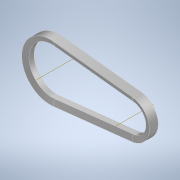
# Autodesk Inventor part: Klapp_Keilriemen
Saved by Autodesk Inventor 2021 (Build 250183000, 183)
## iProperties
CustomPartVersion: 1
Created: 2021-01-13
Part Number: Klapp_Keilriemen
Material: Rubber
Document SubType Name: Modeling
Designer: Jaro Machnow
Density: 0.93 g/cm^3
Appearance: Rubber - Black - Version 1.1
Author: Jaro Machnow
Autodesk Inventor part; units mm, degrees
ref_plane "YZ Plane" through (0, 0, 0) normal (1, 0, 0) x (0, 1, 0)
ref_plane "XZ Plane" through (0, 0, 0) normal (0, 1, 0) x (-1, 0, 0)
sketch "Skizzenpfad" plane through (0, 0, 0) normal (0, 0, 1) x (1, 0, 0)
  arc A0 (-98.3681, 14.911) -> (-98.3681, -14.911) centre (-100, 0) ccw
  arc A1 (-52.9542, -9.9406) -> (-52.9542, 9.9406) centre (-54.0422, 0) ccw
  line L0 (-52.9542, -9.9406) -> (-98.3681, -14.911)
  line L1 (-98.3681, 14.911) -> (-52.9542, 9.9406)
  constraints: 4 end point, 4 point on circle, 2 centre point
ref_plane "Querschnittsebene" through (-98.3681, -14.911, 0) normal (0.9941, 0.1088, 0) x (0, 0, 1)
sketch "Querschnitt" plane through (-98.3681, -14.911, 0) normal (0.9941, 0.1088, 0) x (0, 0, 1)
  line L0 (0, 1.2493) -> (0, -1.7507) construction
  line L1 (-2.1, 0) -> (2.1, 0) construction
  line L2 (-2.5547, 1.2493) -> (2.5547, 1.2493)
  line L3 (2.5547, 1.2493) -> (1.4628, -1.7507)
  line L4 (1.4628, -1.7507) -> (-1.4628, -1.7507)
  line L5 (-1.4628, -1.7507) -> (-2.5547, 1.2493)
  point P0 (0, 0)
  point P1 (0, 0)
  point P2 (0, 0)
  dimension "d0" = 4.2
  dimension "d1" = 1.2493
  dimension "d2" = 40
  dimension "d3" = 3
  constraints: 12 end point, 3 midpoint, 2 parallel, 2 point on line, 1 coincident, 1 perpendicular, 1 vertical, 1 other
  measures "d0" distance of L1.start L1.end
  measures "d1" distance between parallel lines of L2 L1
  measures "d2" angle of L5 L3
  measures "d3" distance between parallel lines of L4 L2
sweep "Riemen" add profiles "Querschnitt" path "Skizzenpfad"
equation "\"d0\" = da_Bw"
equation "\"d1\" = da_Hw"
equation "\"d2\" = da_Alfa"
equation "\"d3\" = da_H"
equation "\"da_Alfa\" = 40deg"
equation "\"da_H\" = 3"
equation "\"da_Bw\" = 4.2"
equation "\"da_Hw\" = 1.2493"
body "Solid1"
